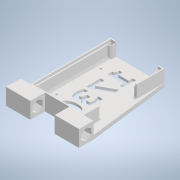
# Autodesk Inventor part: Part2
Saved by Autodesk Inventor 2020 (Build 240168000, 168)
## iProperties
Created: 2020-01-18
Part Number: Part2
Material: Generic
Document SubType Name: Modeling
Designer: Chris Gerth
Density: 1 g/cm^3
Appearance: Default
Author: Chris Gerth
Autodesk Inventor part; units mm, degrees
ref_plane "YZ Plane" through (0, 0, 0) normal (1, 0, 0) x (0, 1, 0)
ref_plane "XZ Plane" through (0, 0, 0) normal (0, 1, 0) x (-1, 0, 0)
ref_plane "XY Plane" through (0, 0, 0) normal (0, 0, 1) x (1, 0, 0)
sketch "Sketch1" plane through (0, 0, 0) normal (0, 1, 0) x (-1, 0, 0)
  line L0 (0, 0) -> (70, 0)
  line L1 (70, 0) -> (70, 105)
  line L2 (70, 105) -> (0, 105)
  line L3 (0, 105) -> (0, 0)
  dimension "d0" = 70
  dimension "d1" = 105
  constraints: 8 end point, 2 parallel, 1 horizontal, 1 perpendicular
  measures "d0" distance of L2.end L1.end
  measures "d1" distance of L1.end L0.end
extrude "Extrusion1" add sketch "Sketch1" along normal blind 3.175
sketch "Sketch2" plane through (0, 3.175, 0) normal (0, 1, 0) x (1, 0, 0)
  line L0 (-70, 0) -> (-70, -105) projected
  line L1 (0, -105) -> (0, 0) projected
  line L2 (-70, -105) -> (0, -105)
  line L3 (0, -105) -> (0, 0)
  line L4 (0, 0) -> (-7, 0)
  line L5 (-70, 0) -> (-70, -105)
  line L6 (-66.825, -101.825) -> (-3.175, -101.825)
  line L7 (-3.175, -101.825) -> (-3.175, -3.175)
  line L8 (-3.175, -3.175) -> (-66.825, -3.175)
  line L9 (-66.825, -3.175) -> (-66.825, -101.825)
  line L10 (0, 0) -> (-70, 0) projected
  line L11 (-63, -3.175) -> (-7, -3.175)
  line L12 (-7, -3.175) -> (-7, 0)
  line L13 (-7, 0) -> (-63, 0)
  line L14 (-63, 0) -> (-63, -3.175)
  line L15 (-7, 0) -> (-63, 0)
  line L16 (-63, 0) -> (-70, 0)
  point P0 (-6.0913, 0)
  point P1 (-7, -3.175)
  point P2 (-62.0913, 0)
  point P3 (-7, -3.175)
  dimension "d4" = 3.175
  dimension "d5" = 3.175
  dimension "d6" = 3.175
  dimension "d7" = 3.175
  dimension "d8" = 56
  constraints: 28 end point, 12 parallel, 3 horizontal, 3 perpendicular, 2 point on line, 1 collinear
  measures "d4" distance between parallel lines of L4 L8
  measures "d5" distance between parallel lines of L0 L9
  measures "d6" distance between parallel lines of L2 L6
  measures "d7" distance between parallel lines of L1 L7
  measures "d8" distance between parallel lines of L12 L14
extrude "Extrusion2" add sketch "Sketch2" along normal blind 15 contours L10 L14 L8 L9 L6 L7 L12 L4 L1 L2 L0
sketch "Sketch3" plane through (0, 3.175, 0) normal (0, 1, 0) x (1, 0, 0)
  circle A0 centre (-10.5, -81.5) radius 1.375
  line L0 (-7, 0) -> (-63, 0) projected
  line L1 (-7, 0) -> (-7, -3.175) projected
  circle A1 centre (-59.5, -81.5) radius 1.3716
  circle A2 centre (-59.5, -23.5) radius 1.3716
  circle A3 centre (-10.5, -23.5118) radius 1.3716
  point P0 (0, 0)
  dimension "d11" = 2.75
  dimension "d12" = 81.5
  dimension "d13" = 3.5
  dimension "d14" = 2.7432
  dimension "d15" = 49
  dimension "d16" = 81.5
  dimension "d17" = 2.7432
  dimension "d18" = 58
  dimension "d19" = 49
  dimension "d20" = 2.7432
  dimension "d21" = 57.9882
  constraints: 4 centre point
  measures "d11" diameter of A0
  measures "d12" distance from line of L0 A0.centre
  measures "d13" distance from line of L1 A0.centre
  measures "d14" diameter of A1
  measures "d15" distance of A0.centre A1.centre
  measures "d16" distance from line of L0 A1.centre
  measures "d17" diameter of A2
  measures "d18" distance of A2.centre A1.centre
  measures "d19" horizontal distance of A0.centre A2.centre
  measures "d20" diameter of A3
  measures "d21" distance of A3.centre A0.centre
extrude "Extrusion3" cut sketch "Sketch3" against normal blind 20
sketch "Sketch4" plane through (0, 18.175, 0) normal (0, 1, 0) x (1, 0, 0)
  line L0 (-70, 0) -> (-70, -105) projected
  line L1 (-70, -105) -> (0, -105)
  line L2 (0, -105) -> (0, 0)
  line L3 (0, 0) -> (-70, 0)
  line L4 (-70, 0) -> (-70, -105)
  line L5 (-68.4125, -103.4125) -> (-1.5875, -103.4125)
  line L6 (-1.5875, -103.4125) -> (-1.5875, -1.5875)
  line L7 (-1.5875, -1.5875) -> (-68.4125, -1.5875)
  line L8 (-68.4125, -1.5875) -> (-68.4125, -103.4125)
  line L9 (-7, -3.175) -> (-7, 0) projected
  line L10 (-7, -1.5875) -> (-7, 0)
  line L11 (-63, 0) -> (-63, -3.175) projected
  line L12 (-63, -1.5875) -> (-63, 0)
  point P0 (-7, -1.5875)
  point P1 (-63, -1.5875)
  dimension "d24" = 1.5875
  dimension "d25" = 1.5875
  dimension "d26" = 1.5875
  dimension "d27" = 1.5875
  constraints: 20 end point, 4 parallel, 2 collinear, 2 horizontal, 2 midpoint, 2 perpendicular
  measures "d24" distance between parallel lines of L8 L0
  measures "d25" distance between parallel lines of L1 L5
  measures "d26" distance between parallel lines of L3 L7
  measures "d27" distance between parallel lines of L2 L6
extrude "Extrusion4" add sketch "Sketch4" along normal blind 3.175 contours L3 L11 L7 L8 L5 L6 L9 L2 L1 L0
sketch "Sketch6" plane through (0, 0, 0) normal (0, -1, 0) x (1, 0, 0)
  line L0 (-49.4418, 10.135) -> (-49.4418, 40.3473) construction
  line L1 (-49.4418, 40.3473) -> (25.087, 40.3473) construction
  line L2 (25.087, 40.3473) -> (25.087, 10.135) construction
  line L3 (25.087, 10.135) -> (-49.4418, 10.135) construction
  line L4 (-23.5067, 30.245) -> (-23.5067, 13.4695)
  line L5 (-23.5067, 13.4695) -> (-27.9321, 13.4695)
  line L6 (-27.9321, 13.4695) -> (-27.9321, 18.8212)
  line L7 (-27.9321, 18.8212) -> (-41.3731, 18.8212)
  line L8 (-41.3731, 18.8212) -> (-41.3731, 13.4695)
  line L9 (-41.3731, 13.4695) -> (-45.5104, 13.4695)
  spline S0 degree 2 poles (-45.5104, 13.4695) (-45.5104, 14.6428) (-45.8191, 16.9687) (-46.1485, 17.6685) knots 0 0 0 1 2 2 2
  spline S1 degree 2 poles (-46.1485, 17.6685) (-46.5601, 18.4713) (-47.9392, 19.377) (-48.9684, 19.4593) knots 0 0 0 1 2 2 2
  line L10 (-48.9684, 19.4593) -> (-48.9684, 25.0168)
  line L11 (-48.9684, 25.0168) -> (-27.9321, 25.0168)
  line L12 (-27.9321, 25.0168) -> (-27.9321, 30.245)
  line L13 (-27.9321, 30.245) -> (-23.5067, 30.245)
  line L14 (-43.8637, 53.0721) -> (-23.5067, 42.2246)
  line L15 (-23.5067, 42.2246) -> (-23.5067, 35.1439)
  line L16 (-23.5067, 35.1439) -> (-44.1107, 46.4854)
  line L17 (-44.1107, 46.4854) -> (-44.1107, 34.3823)
  line L18 (-44.1107, 34.3823) -> (-48.9067, 34.3823)
  line L19 (-48.9067, 34.3823) -> (-48.9067, 53.0721)
  line L20 (-48.9067, 53.0721) -> (-43.8637, 53.0721)
  spline S2 degree 2 poles (-31.2049, 75.2405) (-29.3318, 75.2405) (-26.2648, 73.8614) (-25.1945, 72.5235) knots 0 0 0 1 2 2 2
  spline S3 degree 2 poles (-25.1945, 72.5235) (-24.1242, 71.1856) (-22.9715, 67.5423) (-22.9715, 64.9282) knots 0 0 0 1 2 2 2
  spline S4 degree 2 poles (-22.9715, 64.9282) (-22.9715, 61.9642) (-23.9595, 57.724) (-24.577, 56.386) knots 0 0 0 1 2 2 2
  line L21 (-24.577, 56.386) -> (-30.0934, 56.386)
  line L22 (-30.0934, 56.386) -> (-30.0934, 57.0036)
  spline S5 degree 2 poles (-30.0934, 57.0036) (-29.2083, 58.4032) (-27.8909, 62.17) (-27.8909, 63.7343) knots 0 0 0 1 2 2 2
  spline S6 degree 2 poles (-27.8909, 63.7343) (-27.8909, 64.6606) (-28.2203, 66.8219) (-28.7554, 67.5629) knots 0 0 0 1 2 2 2
  spline S7 degree 2 poles (-28.7554, 67.5629) (-29.1877, 68.1392) (-30.4433, 68.839) (-31.5754, 68.839) knots 0 0 0 1 2 2 2
  spline S8 degree 2 poles (-31.5754, 68.839) (-32.7075, 68.839) (-33.9219, 67.851) (-34.2101, 67.0277) knots 0 0 0 1 2 2 2
  spline S9 degree 2 poles (-34.2101, 67.0277) (-34.4982, 66.2044) (-34.56, 63.9196) (-34.56, 63.0345) knots 0 0 0 1 2 2 2
  line L23 (-34.56, 63.0345) -> (-34.56, 61.9436)
  line L24 (-34.56, 61.9436) -> (-39.0266, 61.9436)
  line L25 (-39.0266, 61.9436) -> (-39.0266, 62.9522)
  spline S10 degree 2 poles (-39.0266, 62.9522) (-39.0266, 64.1048) (-39.2324, 66.0603) (-39.5412, 66.7395) knots 0 0 0 1 2 2 2
  spline S11 degree 2 poles (-39.5412, 66.7395) (-39.8705, 67.4188) (-41.0232, 68.1804) (-42.0112, 68.1804) knots 0 0 0 1 2 2 2
  spline S12 degree 2 poles (-42.0112, 68.1804) (-42.7934, 68.1804) (-43.7608, 67.46) (-44.0284, 66.9454) knots 0 0 0 1 2 2 2
  spline S13 degree 2 poles (-44.0284, 66.9454) (-44.3371, 66.3279) (-44.543, 64.6812) (-44.543, 64.1048) knots 0 0 0 1 2 2 2
  spline S14 degree 2 poles (-44.543, 64.1048) (-44.543, 63.1786) (-44.1107, 61.2232) (-43.7608, 60.3175) knots 0 0 0 1 2 2 2
  spline S15 degree 2 poles (-43.7608, 60.3175) (-43.4932, 59.5971) (-42.6287, 58.0327) (-42.4023, 57.6622) knots 0 0 0 1 2 2 2
  line L26 (-42.4023, 57.6622) -> (-42.4023, 57.1271)
  line L27 (-42.4023, 57.1271) -> (-47.8363, 57.1271)
  spline S16 degree 2 poles (-47.8363, 57.1271) (-48.3921, 58.4444) (-49.4418, 62.8904) (-49.4418, 65.2164) knots 0 0 0 1 2 2 2
  spline S17 degree 2 poles (-49.4418, 65.2164) (-49.4418, 67.4805) (-48.6597, 70.8151) (-47.8981, 71.9883) knots 0 0 0 1 2 2 2
  spline S18 degree 2 poles (-47.8981, 71.9883) (-47.0953, 73.2851) (-44.6253, 74.5818) (-43.0815, 74.5818) knots 0 0 0 1 2 2 2
  spline S19 degree 2 poles (-43.0815, 74.5818) (-40.8997, 74.5818) (-37.6475, 72.0707) (-37.1741, 70.0123) knots 0 0 0 1 2 2 2
  line L28 (-37.1741, 70.0123) -> (-36.9271, 70.0123)
  spline S20 degree 2 poles (-36.9271, 70.0123) (-36.8036, 70.918) (-36.1449, 72.647) (-35.4039, 73.4703) knots 0 0 0 1 2 2 2
  spline S21 degree 2 poles (-35.4039, 73.4703) (-34.7452, 74.2319) (-32.6457, 75.2405) (-31.2049, 75.2405) knots 0 0 0 1 2 2 2
  spline S22 degree 2 poles (-32.1517, 97.9852) (-28.1379, 97.9852) (-22.9715, 92.9011) (-22.9715, 88.4551) knots 0 0 0 1 2 2 2
  spline S23 degree 2 poles (-22.9715, 88.4551) (-22.9715, 86.2321) (-24.2477, 82.7535) (-25.5033, 81.539) knots 0 0 0 1 2 2 2
  spline S24 degree 2 poles (-25.5033, 81.539) (-26.9647, 80.0982) (-31.596, 78.5544) (-34.8276, 78.5544) knots 0 0 0 1 2 2 2
  spline S25 degree 2 poles (-34.8276, 78.5544) (-38.1621, 78.5544) (-43.3491, 79.9953) (-45.3457, 81.6214) knots 0 0 0 1 2 2 2
  spline S26 degree 2 poles (-45.3457, 81.6214) (-47.2394, 83.1651) (-49.3801, 88.1875) (-49.3801, 91.6249) knots 0 0 0 1 2 2 2
  spline S27 degree 2 poles (-49.3801, 91.6249) (-49.3801, 92.8805) (-49.0507, 95.3917) (-48.9478, 95.8446) knots 0 0 0 1 2 2 2
  line L29 (-48.9478, 95.8446) -> (-43.9666, 95.8446)
  line L30 (-43.9666, 95.8446) -> (-43.9666, 95.3917)
  spline S28 degree 2 poles (-43.9666, 95.3917) (-44.193, 94.9389) (-44.7488, 92.8805) (-44.7488, 91.5632) knots 0 0 0 1 2 2 2
  spline S29 degree 2 poles (-44.7488, 91.5632) (-44.7488, 88.5786) (-41.5995, 85.3264) (-38.6767, 84.9353) knots 0 0 0 1 2 2 2
  spline S30 degree 2 poles (-38.6767, 84.9353) (-39.4794, 86.1909) (-40.4263, 88.7638) (-40.4263, 90.3899) knots 0 0 0 1 2 2 2
  spline S31 degree 2 poles (-40.4263, 90.3899) (-40.4263, 91.769) (-39.6853, 94.1773) (-38.9854, 95.1036) knots 0 0 0 1 2 2 2
  spline S32 degree 2 poles (-38.9854, 95.1036) (-37.9768, 96.4209) (-34.7041, 97.9852) (-32.1517, 97.9852) knots 0 0 0 1 2 2 2
  spline S33 degree 2 poles (-28.3232, 90.5546) (-28.9407, 91.0486) (-30.3815, 91.5838) (-31.843, 91.5838) knots 0 0 0 1 2 2 2
  spline S34 degree 2 poles (-31.843, 91.5838) (-33.078, 91.5838) (-34.6835, 90.9663) (-35.1569, 90.4105) knots 0 0 0 1 2 2 2
  spline S35 degree 2 poles (-35.1569, 90.4105) (-35.6509, 89.8342) (-36.0008, 88.4139) (-36.0008, 87.6112) knots 0 0 0 1 2 2 2
  spline S36 degree 2 poles (-36.0008, 87.6112) (-36.0008, 86.9319) (-35.6509, 85.5322) (-35.4039, 84.9147) knots 0 0 0 1 2 2 2
  spline S37 degree 2 poles (-35.4039, 84.9147) (-35.2392, 84.9147) (-34.4571, 84.8736) (-33.8601, 84.8736) knots 0 0 0 1 2 2 2
  spline S38 degree 2 poles (-33.8601, 84.8736) (-31.6577, 84.8736) (-29.0024, 85.6352) (-28.3232, 86.2321) knots 0 0 0 1 2 2 2
  spline S39 degree 2 poles (-28.3232, 86.2321) (-27.7674, 86.6643) (-27.294, 87.817) (-27.294, 88.4345) knots 0 0 0 1 2 2 2
  spline S40 degree 2 poles (-27.294, 88.4345) (-27.294, 88.9491) (-27.8086, 90.1429) (-28.3232, 90.5546) knots 0 0 0 1 2 2 2
  point P0 (0, 0)
  constraints: 2 other
extrude "Extrusion5" cut sketch "Sketch6" against normal blind 6.604
sketch "Sketch7" plane through (0, 0, 0) normal (0, -1, 0) x (1, 0, 0)
  line L0 (-70, 0) -> (-70, 105) projected
  line L1 (-70, 0) -> (-82.7, 0)
  line L2 (-82.7, 0) -> (-82.7, 105)
  line L3 (-82.7, 105) -> (-70, 105)
  line L4 (-70, 105) -> (-70, 0)
  line L5 (0, 105) -> (12.7, 105)
  line L6 (12.7, 105) -> (12.7, 0)
  line L7 (12.7, 0) -> (0, 0)
  line L8 (0, 0) -> (0, 105)
  dimension "d32" = 12.7
  dimension "d33" = 12.7
  constraints: 16 end point, 4 parallel, 2 horizontal, 2 perpendicular, 2 point on line
  measures "d32" distance of L2.end L3.end
  measures "d33" distance between parallel lines of L6 L8
extrude "Extrusion6" add sketch "Sketch7" against normal blind 5.08
sketch "Sketch8" plane through (0, 0, 0) normal (0, -1, 0) x (1, 0, 0)
  line L0 (-41.0023, 87.4584) -> (-21.5012, 87.4584)
  line L1 (-21.5012, 87.4584) -> (-21.5012, 89.834)
  line L2 (-21.5012, 89.834) -> (-41.0023, 89.834)
  line L3 (-41.0023, 89.834) -> (-41.0023, 87.4584)
  point P0 (0, 0)
  constraints: 8 end point, 2 parallel, 1 horizontal, 1 perpendicular
extrude "Extrusion7" add sketch "Sketch8" against normal blind 3.175
sketch "Sketch9" plane through (0, 3.175, 0) normal (0, 1, 0) x (1, 0, 0)
  line L0 (-66.825, -3.175) -> (-66.825, -101.825) projected
  line L1 (-66.825, -3.175) -> (-63, -3.175) projected
  arc A0 (-66.825, -7) -> (-63, -3.175) centre (-66.825, -3.175) ccw
  line L2 (-7, -3.175) -> (-3.175, -3.175) projected
  line L3 (-7, -1.5875) -> (-7, -3.175) projected
  arc A1 (-7, -3.175) -> (-3.175, -7) centre (-3.175, -3.175) ccw
  line L4 (-66.825, -101.825) -> (-66.825, -3.175) projected
  arc A2 (-63, -101.825) -> (-66.825, -98) centre (-66.825, -101.825) ccw
  line L5 (-3.175, -101.825) -> (-66.825, -101.825) projected
  line L6 (-3.175, -3.175) -> (-3.175, -101.825) projected
  arc A3 (-3.175, -98) -> (-7, -101.825) centre (-3.175, -101.825) ccw
  point P0 (0, 0)
  point P1 (-66.825, -7)
  constraints: 8 point on circle, 4 centre point, 2 equal radius, 2 point on line, 1 coincident
extrude "Extrusion8" add sketch "Sketch9" along normal up to surface (15 mm away)
sketch "Sketch10" plane through (0, 18.175, 0) normal (0, 1, 0) x (1, 0, 0)
  circle A0 centre (-66.19, -3.81) radius 2.159
  line L0 (-63, 0) -> (-70, 0) projected
  circle A1 centre (-3.81, -3.81) radius 2.159
  line L1 (0, 0) -> (-7, 0) projected
  line L2 (-70, 0) -> (-70, -105) projected
  line L3 (0, -105) -> (0, 0) projected
  circle A2 centre (-66.19, -101.19) radius 2.159
  circle A3 centre (-3.81, -101.19) radius 2.159
  line L4 (-70, -105) -> (0, -105) projected
  dimension "d40" = 4.318
  dimension "d41" = 3.81
  dimension "d42" = 3.81
  dimension "d43" = 3.81
  dimension "d44" = 3.81
  dimension "d47" = 3.81
  dimension "d48" = 3.81
  dimension "d49" = 3.81
  dimension "d50" = 3.81
  constraints: 4 centre point, 3 equal radius
  measures "d40" diameter of A0
  measures "d41" distance from line of L0 A0.centre
  measures "d42" distance from line of L1 A1.centre
  measures "d43" distance from line of L2 A0.centre
  measures "d44" distance from line of L3 A1.centre
  measures "d47" distance from line of L2 A2.centre
  measures "d48" distance from line of L4 A2.centre
  measures "d49" distance from line of L4 A3.centre
  measures "d50" distance from line of L3 A3.centre
extrude "Extrusion9" cut sketch "Sketch10" against normal through all
fillet "Fillet2" radius 3.175 5 edges at (-3.175, 3.175, 52.5) (-35, 3.175, 101.825) (-5.8797, 3.175, 99.1203) (-66.825, 3.175, 52.5) (-64.1203, 3.175, 99.1203)
chamfer "Chamfer1" distance 1.5875 angle 45 4 edges at (-5.969, 0, 3.81) (-68.349, 0, 3.81) (-68.349, 0, 101.19) (-5.969, 0, 101.19)
sketch "Sketch12" plane through (0, 21.35, 0) normal (0, 1, 0) x (1, 0, 0)
  line L0 (7.2555, -84.8769) -> (-9.0587, -84.8769)
  line L1 (-9.0587, -84.8769) -> (-9.0587, -36.1059)
  line L2 (-9.0587, -36.1059) -> (7.2555, -36.1059)
  line L3 (7.2555, -36.1059) -> (7.2555, -84.8769)
  point P0 (0, 0)
  constraints: 8 end point, 2 parallel, 1 horizontal, 1 perpendicular
extrude "Extrusion10" cut sketch "Sketch12" against normal up to surface (16.27 mm away)
fillet "Fillet3" radius 3.175 2 edges at (-1.72, 5.08, 36.1059) (-1.72, 5.08, 84.8769)
sketch "Sketch13" plane through (12.7, 0, 105) normal (1, 0, 0) x (0, 0, -1)
  line L0 (0, 21.35) -> (-19.05, 21.35)
  line L1 (-19.05, 21.35) -> (-19.05, 0)
  line L2 (-19.05, 0) -> (0, 0)
  line L3 (0, 0) -> (0, 21.35)
  point P0 (105, 0)
  dimension "d61" = 19.05
  constraints: 8 end point, 2 parallel, 1 horizontal, 1 perpendicular
  measures "d61" distance of L2.end L1.end
extrude "Extrusion11" add sketch "Sketch13" against normal up to surface (95.4 mm away)
sketch "Sketch14" plane through (-82.7, 0, 0) normal (-1, 0, 0) x (0, 0, 1)
  line L0 (120.875, 6.9145) -> (114.398, 3.175)
  line L1 (114.398, 3.175) -> (107.921, 6.9145)
  line L2 (107.921, 6.9145) -> (107.921, 14.3935)
  line L3 (107.921, 14.3935) -> (114.398, 18.133)
  line L4 (114.398, 18.133) -> (120.875, 14.3935)
  line L5 (120.875, 14.3935) -> (120.875, 6.9145)
  line L6 (124.05, 21.35) -> (124.05, 0) projected
  line L7 (124.05, 0) -> (0, 0) projected
  point P0 (114.398, 10.654)
  dimension "d64" = 12.954
  dimension "d65" = 3.175
  dimension "d66" = 3.175
  constraints: 12 end point, 1 parallel, 13 other
  measures "d64" distance between parallel lines of L5 L2
  measures "d65" distance from line of L7 L0.end
  measures "d66" distance between parallel lines of L6 L5
extrude "Extrusion12" cut sketch "Sketch14" against normal up to surface (95.4 mm away)
sketch "Sketch15" plane through (12.7, 0, 124.05) normal (0, 0, 1) x (1, 0, 0)
  line L0 (0, 21.35) -> (-95.4, 21.35) projected
  line L1 (0, 0) -> (-95.4, 0) projected
  line L2 (-63.65, 21.35) -> (-31.75, 21.35)
  line L3 (-31.75, 21.35) -> (-31.75, 0)
  line L4 (-31.75, 0) -> (-63.65, 0)
  line L5 (-63.65, 0) -> (-63.65, 21.35)
  line L6 (0, 21.35) -> (0, 0) projected
  line L7 (-95.4, 21.35) -> (-95.4, 0) projected
  point P0 (-12.7, 0)
  point P1 (-63.65, 0)
  dimension "d69" = 31.75
  dimension "d70" = 31.75
  constraints: 8 end point, 2 parallel, 2 point on line, 1 horizontal, 1 perpendicular
  measures "d69" distance between parallel lines of L6 L3
  measures "d70" distance between parallel lines of L5 L7
extrude "Extrusion13" cut sketch "Sketch15" against normal up to surface (19.05 mm away) contours L3 L1 L5 L0
sketch "Sketch16" plane through (0, 5.08, 0) normal (0, 1, 0) x (1, 0, 0)
  line L0 (12.7, -124.05) -> (12.7, 0) projected
  line L1 (12.7, 0) -> (0, 0) projected
  line L2 (12.7, -105.0352) -> (0, 0)
  line L3 (0, 0) -> (12.7, 0)
  line L4 (0, -105) -> (12.7, -105) projected
  line L5 (12.7, 0) -> (12.7, -105)
  line L6 (-82.7, -105) -> (-70, -105) projected
  line L7 (-82.7, -105) -> (-82.7, 0)
  line L8 (-82.7, 0) -> (-70, 0)
  line L9 (-70, 0) -> (-82.7, -105)
  point P0 (12.6957, -105)
  constraints: 12 end point, 2 perpendicular, 1 collinear, 1 point on line, 1 vertical
extrude "Extrusion14" cut sketch "Sketch16" against normal blind 25.4 contours L4 L2 L1 L0 | L7 L8 L9
body "Solid1"
